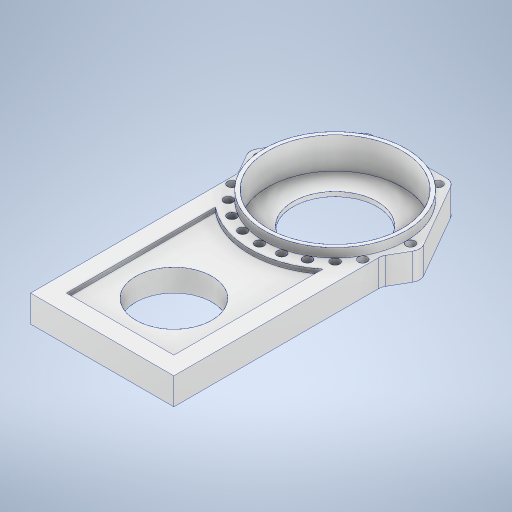
# Autodesk Inventor part: PatronDerzavka
Saved by Autodesk Inventor 2024 (Build 280153000, 153)
## iProperties
Created: 2023-08-22
Part Number: PatronDerzavka
Material: Aluminum 6061
Document SubType Name: Modeling
Designer: KirikDK
Density: 2.7 g/cm^3
Appearance: Aluminum - Flat
Mass: 1780.3 g
Surface Area: 1365.77 cm^2
Volume: 659.372 cm^3
Author: KirikDK
Autodesk Inventor part; units mm, degrees
ref_plane "YZ Plane" through (0, 0, 0) normal (1, 0, 0) x (0, 1, 0)
ref_plane "XZ Plane" through (0, 0, 0) normal (0, 1, 0) x (-1, 0, 0)
ref_plane "XY Plane" through (0, 0, 0) normal (0, 0, 1) x (1, 0, 0)
sketch "Sketch1" plane through (0, 0, 0) normal (0, 1, 0) x (-1, 0, 0)
  line L0 (24.2857, 221.4286) -> (-135.7143, 221.4286)
  line L1 (-135.7143, 221.4286) -> (-135.7143, -28.5714)
  line L2 (-135.7143, -28.5714) -> (24.2857, -28.5714)
  line L3 (24.2857, -28.5714) -> (24.2857, 221.4286)
  circle A0 centre (-55.7143, -38.5714) radius 80
  line L4 (24.2857, -28.5714) -> (24.2857, -38.5714)
  line L5 (-135.7143, -28.5714) -> (-135.7143, -38.5714)
  point P0 (0, 0)
  dimension "d0" = 250
  dimension "d1" = 160
  dimension "d2" = 160
  dimension "d8" = 10
  constraints: 12 end point, 2 parallel, 2 point on circle, 1 centre point, 1 horizontal, 1 perpendicular, 1 tangent, 1 vertical
  measures "d0" distance of L2.end L0.start
  measures "d1" distance of L0.start L0.end
  measures "d2" diameter of A0
  measures "d8" distance from line of A0.centre L2
extrude "Extrusion1" add sketch "Sketch1" along normal blind 30
sketch "Sketch2" plane through (0, 30, 0) normal (0, 1, 0) x (1, 0, 0)
  arc A0 (135.7143, 38.5714) -> (-24.2857, 38.5714) centre (55.7143, 38.5714) ccw projected
  circle A1 centre (55.7143, 38.5714) radius 75
  point P0 (0, 0)
  dimension "d5" = 150
  constraints: 1 centre point, 1 coincident
  measures "d5" diameter of A1
extrude "Extrusion2" cut sketch "Sketch2" against normal blind 40
sketch "Sketch3" plane through (0, 30, 0) normal (0, 1, 0) x (1, 0, 0)
  circle A0 centre (55.7143, 38.5714) radius 75 projected
  circle A1 centre (55.7143, 38.5714) radius 75
  line L0 (152, 38.5714) -> (103.8571, -44.8144)
  line L1 (103.8571, -44.8144) -> (7.5714, -44.8144)
  line L2 (7.5714, -44.8144) -> (-40.5714, 38.5714)
  line L3 (-40.5714, 38.5714) -> (7.5714, 121.9573)
  line L4 (7.5714, 121.9573) -> (103.8571, 121.9573)
  line L5 (103.8571, 121.9573) -> (152, 38.5714)
  line L6 (140, 38.5714) -> (97.8571, -34.4221)
  line L7 (97.8571, -34.4221) -> (13.5714, -34.4221)
  line L8 (13.5714, -34.4221) -> (-28.5714, 38.5714)
  line L9 (-28.5714, 38.5714) -> (13.5714, 111.565)
  line L10 (13.5714, 111.565) -> (97.8571, 111.565)
  line L11 (97.8571, 111.565) -> (140, 38.5714)
  circle A2 centre (140, 38.5714) radius 5
  circle A3 centre (97.8571, 111.565) radius 5
  circle A4 centre (13.5714, 111.565) radius 5
  circle A5 centre (-28.5714, 38.5714) radius 5
  circle A6 centre (13.5714, -34.4221) radius 5
  circle A7 centre (97.8571, -34.4221) radius 5
  point P0 (0, 0)
  dimension "d15" = 360
  constraints: 24 end point, 7 centre point, 4 coincident, 39 other
sketch "Sketch4" plane through (0, 0, 0) normal (0, -1, 0) x (1, 0, 0)
  circle A0 centre (55.7143, -38.5714) radius 75 projected
  circle A1 centre (55.7143, -38.5714) radius 75
  circle A2 centre (55.7143, -38.5714) radius 47
  dimension "d9" = 94
  dimension "d10" = 150
  constraints: 2 centre point, 2 coincident
  measures "d9" diameter of A2
  measures "d10" diameter of A1
extrude "Extrusion3" add sketch "Sketch4" against normal blind 5
sketch "Sketch5" plane through (0, 30, 0) normal (0, 1, 0) x (1, 0, 0)
  circle A0 centre (55.7143, 38.5714) radius 75
  circle A1 centre (55.7143, 38.5714) radius 75
  line L0 (152, 38.5714) -> (103.8571, -44.8144)
  line L1 (103.8571, -44.8144) -> (7.5714, -44.8144)
  line L2 (7.5714, -44.8144) -> (-40.5714, 38.5714)
  line L3 (-40.5714, 38.5714) -> (7.5714, 121.9573)
  line L4 (7.5714, 121.9573) -> (103.8571, 121.9573)
  line L5 (103.8571, 121.9573) -> (152, 38.5714)
  line L6 (140, 38.5714) -> (97.8571, -34.4221)
  line L7 (97.8571, -34.4221) -> (13.5714, -34.4221)
  line L8 (13.5714, -34.4221) -> (-28.5714, 38.5714)
  line L9 (-28.5714, 38.5714) -> (13.5714, 111.565)
  line L10 (13.5714, 111.565) -> (97.8571, 111.565)
  line L11 (97.8571, 111.565) -> (140, 38.5714)
  circle A2 centre (140, 38.5714) radius 5
  circle A3 centre (97.8571, 111.565) radius 5
  circle A4 centre (13.5714, 111.565) radius 5
  circle A5 centre (-28.5714, 38.5714) radius 5
  circle A6 centre (13.5714, -34.4221) radius 5
  circle A7 centre (97.8571, -34.4221) radius 5
  arc A8 (135.7143, 38.5714) -> (-24.2857, 38.5714) centre (55.7143, 38.5714) ccw projected
  circle A9 centre (55.7143, 38.5714) radius 2.2469
  point P0 (0, 0)
  point P1 (0, 0)
  dimension "d19" = 360
  constraints: 24 end point, 9 centre point, 5 coincident, 39 other
extrude "Extrusion4" cut sketch "Sketch5" against normal blind 30 contours A2 L11 L6 | L6 L11 A2 | A7 L7 L6 | L6 L7 A7 | A3 A8 L10 L11 | L11 L10 A3 | A3 A8 | A6 L8 L7 | L7 L8 A6 | A4 A8 L9 L10 | L10 L9 A4 | A4 A8 | A5 L9 L8 | L8 L9 A5
extrude "Extrusion5" add sketch "Sketch3" against normal blind 30 contours A0 L11 A2 L6 | A0 L10 A3 L11 | L6 A7 L7 A0 | A0 L9 A4 L10 | L7 A6 L8 A0 | A0 L8 A5 L9 | L0 L1 L2 L3 L4 L5
fillet "Fillet1" radius 12 6 edges at (103.8571, 15, -121.9573) (152, 15, -38.5714) (7.5714, 15, -121.9573) (-40.5714, 15, -38.5714) (-24.2857, 15, -10.3637) (135.7143, 15, -10.3637)
sketch "Sketch6" plane through (0, 30, 0) normal (0, 1, 0) x (1, 0, 0)
  circle A0 centre (13.5714, 111.565) radius 5 projected
  circle A1 centre (97.8571, 111.565) radius 5 projected
  circle A2 centre (-28.5714, 38.5714) radius 5 projected
  circle A3 centre (140, 38.5714) radius 5 projected
  circle A4 centre (55.7143, 38.5714) radius 75 projected
  circle A5 centre (97.8571, -34.4221) radius 5 projected
  circle A6 centre (13.5714, -34.4221) radius 5 projected
  arc A7 (-37.1073, 44.5714) -> (-37.1073, 32.5714) centre (-26.715, 38.5714) ccw projected
  line L0 (-37.1073, 32.5714) -> (-25.8934, 13.1484) projected
  arc A8 (-24.2857, 7.1484) -> (-25.8934, 13.1484) centre (-36.2857, 7.1484) ccw projected
  line L1 (-24.2857, 7.1484) -> (-24.2857, -221.4286) projected
  line L2 (-24.2857, -221.4286) -> (135.7143, -221.4286) projected
  line L3 (135.7143, -221.4286) -> (135.7143, 7.1484) projected
  arc A9 (137.322, 13.1484) -> (135.7143, 7.1484) centre (147.7143, 7.1484) ccw projected
  line L4 (137.322, 13.1484) -> (148.5359, 32.5714) projected
  arc A10 (148.5359, 32.5714) -> (148.5359, 44.5714) centre (138.1436, 38.5714) ccw projected
  line L5 (148.5359, 44.5714) -> (107.3212, 115.9573) projected
  arc A11 (107.3212, 115.9573) -> (96.9289, 121.9573) centre (96.9289, 109.9573) ccw projected
  line L6 (96.9289, 121.9573) -> (14.4996, 121.9573) projected
  arc A12 (14.4996, 121.9573) -> (4.1073, 115.9573) centre (14.4996, 109.9573) ccw projected
  line L7 (4.1073, 115.9573) -> (-37.1073, 44.5714) projected
  line L8 (-4.2857, -201.4286) -> (-4.2857, 7.1484)
  arc A13 (-4.2857, 7.1484) -> (-8.5729, 23.1484) centre (-36.2857, 7.1484) ccw
  line L9 (-8.5729, 23.1484) -> (-17.4774, 38.5714)
  line L10 (-17.4774, 38.5714) -> (19.1184, 101.9573)
  line L11 (19.1184, 101.9573) -> (92.3101, 101.9573)
  line L12 (92.3101, 101.9573) -> (128.906, 38.5714)
  line L13 (128.906, 38.5714) -> (120.0015, 23.1484)
  arc A14 (120.0015, 23.1484) -> (115.7143, 7.1484) centre (147.7143, 7.1484) ccw
  line L14 (115.7143, 7.1484) -> (115.7143, -201.4286)
  line L15 (115.7143, -201.4286) -> (-4.2857, -201.4286)
  circle A15 centre (55.7143, 38.5714) radius 95
  point P0 (0, 0)
  point P1 (115.7143, -35.0832)
  point P2 (-4.2857, -35.0832)
  dimension "d25" = 20
  dimension "d26" = 190
  constraints: 16 end point, 4 point on circle, 3 centre point, 1 coincident, 9 other
  measures "d25" distance between parallel lines of L1 L8
  measures "d26" diameter of A15
extrude "Extrusion6" cut sketch "Sketch6" against normal blind 5 contours A15 L14 L15 L8
sketch "Sketch7" plane through (0, 30, 0) normal (0, 1, 0) x (1, 0, 0)
  circle A0 centre (55.7143, 38.5714) radius 75 projected
  circle A1 centre (55.7143, 38.5714) radius 79.2857
  circle A2 centre (-28.5714, 38.5714) radius 5 projected
  circle A3 centre (55.7143, 38.5714) radius 75
  point P0 (0, 0)
  dimension "d29" = 150
  constraints: 2 centre point, 2 coincident, 1 tangent
  measures "d29" diameter of A3
extrude "Extrusion7" add sketch "Sketch7" along normal blind 10 contours A1
sketch "Sketch8" plane through (0, 30, 0) normal (0, 1, 0) x (1, 0, 0)
  circle A0 centre (55.7143, -45.7146) radius 5
  circle A1 centre (55.7143, 38.5714) radius 47 projected
  circle A2 centre (77.5291, -42.8426) radius 5
  circle A3 centre (97.8573, -34.4224) radius 5
  circle A4 centre (115.3135, -21.0278) radius 5
  circle A5 centre (128.7081, -3.5716) radius 5
  circle A6 centre (137.1283, 16.7566) radius 5
  circle A7 centre (140.0003, 38.5714) radius 5
  circle A8 centre (137.1283, 60.3863) radius 5
  circle A9 centre (128.7081, 80.7144) radius 5
  circle A10 centre (115.3135, 98.1706) radius 5
  circle A11 centre (97.8573, 111.5652) radius 5
  circle A12 centre (77.5291, 119.9855) radius 5
  circle A13 centre (55.7143, 122.8574) radius 5
  circle A14 centre (33.8995, 119.9855) radius 5
  circle A15 centre (13.5713, 111.5652) radius 5
  circle A16 centre (-3.8849, 98.1706) radius 5
  circle A17 centre (-17.2795, 80.7144) radius 5
  circle A18 centre (-25.6997, 60.3863) radius 5
  circle A19 centre (-28.5717, 38.5714) radius 5
  circle A20 centre (-25.6997, 16.7566) radius 5
  circle A21 centre (-17.2795, -3.5716) radius 5
  circle A22 centre (-3.8849, -21.0278) radius 5
  circle A23 centre (13.5713, -34.4224) radius 5
  circle A24 centre (33.8995, -42.8426) radius 5
  point P0 (0, 0)
  dimension "d32" = 84.286
  dimension "d35" = 360
  dimension "d39" = 10
  constraints: 24 centre point, 49 other
  measures "d32" distance of A0.centre A1.centre
  measures "d39" diameter of A24
extrude "Extrusion8" cut sketch "Sketch8" against normal blind 35 contours A0 | A2 | A4 | A5 | A21 | A22 | A24
sketch "Sketch9" plane through (0, 25, 0) normal (0, 1, 0) x (1, 0, 0)
  line L0 (135.7143, -221.4286) -> (135.7143, 7.1484) projected
  line L1 (-24.2857, -221.4286) -> (135.7143, -221.4286) projected
  line L2 (-24.2857, 7.1484) -> (-24.2857, -221.4286) projected
  circle A0 centre (55.7143, -141.4286) radius 80
  circle A1 centre (55.7143, -141.4286) radius 42.5
  point P0 (0, 0)
  dimension "d40" = 85
  constraints: 3 tangent, 2 centre point, 1 coincident
  measures "d40" diameter of A1
extrude "Extrusion9" cut sketch "Sketch9" against normal blind 40 contours A1
body "Solid1"
